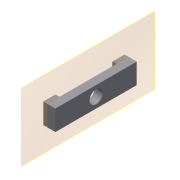
# Autodesk Inventor part: 03_Camera_Clip
Saved by Autodesk Inventor 2019 (Build 230136000, 136)
## iProperties
Created: 2021-09-23
Part Number: 03_Camera_Clip
Material: Generisch
Document SubType Name: Modeling
Designer: Muriel
Density: 1 g/cm^3
Appearance: Vorgabe
Author: Muriel
Autodesk Inventor part; units mm, degrees
ref_plane "YZ Plane" through (0, 0, 0) normal (1, 0, 0) x (0, 1, 0)
ref_plane "XZ Plane" through (0, 0, 0) normal (0, 1, 0) x (-1, 0, 0)
ref_plane "XY Plane" through (0, 0, 0) normal (0, 0, 1) x (1, 0, 0)
ref_plane "Arbeitsebene1" through (-38.5744, -30.9423, 15.3122) normal (1, 0, 0) x (0, 1, 0)
sketch "Skizze1" plane through (-38.5744, -30.9423, 15.3122) normal (1, 0, 0) x (0, 1, 0)
  circle A0 centre (-3.7508, 1.8008) radius 1.4 projected
  line L0 (-1.2508, 11.8008) -> (-6.2508, 11.8008)
  line L1 (-6.2508, 11.8008) -> (-6.2508, -8.1992)
  line L2 (-6.2508, -8.1992) -> (-1.2508, -8.1992)
  line L3 (-1.2508, -8.1992) -> (-1.2508, 11.8008)
  line L4 (-1.2508, 11.8008) -> (-6.2508, -8.1992) construction
  line L5 (-6.2508, 11.8008) -> (-1.2508, -8.1992) construction
  circle A1 centre (-3.7508, 1.8008) radius 1.6
  point P0 (30.9423, -15.3122)
  dimension "d0" = 5
  dimension "d1" = 20
  dimension "d4" = 0.2
  constraints: 12 end point, 2 midpoint, 2 parallel, 1 centre point, 1 horizontal, 1 perpendicular
  measures "d0" distance of L2.end L1.end
  measures "d1" distance of L1.end L0.end
  measures "d4" radial gap between concentric circles of A0 A1
extrude "Extrusion1" add sketch "Skizze1" along normal blind 2 contours L3 L2 L1 L0
sketch "Skizze2" plane through (-38.5744, -30.9423, 15.3122) normal (-1, 0, 0) x (0, 0, 1)
  circle A0 centre (1.8008, -3.7508) radius 1.6 projected
  line L0 (11.8008, -1.2508) -> (11.8008, -6.2508) projected
  line L1 (11.8008, -6.2508) -> (-8.1992, -6.2508) projected
  line L2 (-8.1992, -6.2508) -> (-8.1992, -1.2508) projected
  line L3 (-8.1992, -1.2508) -> (11.8008, -1.2508) projected
  line L4 (-8.1992, -6.2508) -> (-8.1992, -1.2508) projected
  line L5 (11.8008, -6.2508) -> (-8.1992, -6.2508) projected
  line L6 (-8.1992, -1.2508) -> (-5.1992, -1.2508)
  line L7 (-5.1992, -1.2508) -> (-5.1992, -6.2508)
  line L8 (-5.1992, -6.2508) -> (-8.1992, -6.2508)
  line L9 (-8.1992, -6.2508) -> (-8.1992, -1.2508)
  line L10 (-8.1992, -1.2508) -> (11.8008, -1.2508) projected
  line L11 (11.8008, -1.2508) -> (8.8008, -1.2508)
  line L12 (8.8008, -1.2508) -> (8.8008, -6.2508)
  line L13 (8.8008, -6.2508) -> (11.8008, -6.2508)
  line L14 (11.8008, -6.2508) -> (11.8008, -1.2508)
  point P0 (-15.3122, 30.9423)
  dimension "d5" = 3
  dimension "d6" = 3
  constraints: 16 end point, 4 parallel, 2 horizontal, 2 perpendicular, 2 point on line
  measures "d5" distance of L7.end L8.end
  measures "d6" distance of L13.end L12.end
extrude "Extrusion2" add sketch "Skizze2" along normal blind 1 contours L0 L1 L12 L3 | L7 L1 L2 L3
